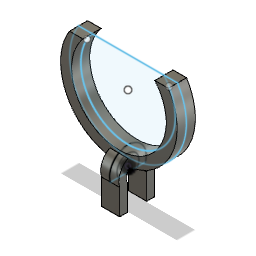
christmas-bell-door-clip-v6 (Autodesk Fusion 360 design; units mm, degrees)
Autodesk Fusion 360 part; units mm, degrees
sketch "Sketch1" plane through (0, 0, 0) normal (0, 0, 1) x (1, 0, 0)
  arc A0 (-11.2804, 24.5601) -> (11.2804, 24.5601) centre (0, 18.0985) ccw
  line L0 (13.5888, 26.545) -> (-13.5888, 26.545)
  arc A1 (-9.8821, 26.545) -> (9.8821, 26.545) centre (0, 18.0985) ccw
  arc A2 (-13.5888, 26.545) -> (13.5888, 26.545) centre (0, 18.0985) ccw
  dimension "d3" = 26
  dimension "d21" = 16
  constraint concentric A0 A1
  constraint horizontal L0
  constraint coincident L0 A1.end
  constraint coincident L0 A1.start
  measures "d3" diameter of A0
  measures "d21" radius of A2
extrude "Extrude1" add sketch "Sketch1" along normal mid plane 5 makes body 1
sketch "Sketch2" plane through (0, 0, 0) normal (1, 0, 0) x (0, 0, -1)
  line L0 (-4.783, -1.457) -> (4.783, -1.457)
  arc A0 (2.6224, -1.457) -> (-2.6224, -1.457) centre (0, 0) ccw
  arc A1 (4.783, -1.457) -> (-4.783, -1.457) centre (0, 0) ccw
  dimension "d9" = 3
  dimension "d10" = 5
  constraint horizontal L0
  constraint concentric A0 A1
  constraint coincident L0 A0.end
  constraint coincident L0 A0.start
  constraint coincident A0.centre A1.centre
  measures "d9" radius of A0
  measures "d10" radius of A1
extrude "Extrude2" add sketch "Sketch2" along normal mid plane 5 separate body contours L0 A0 A1 makes body 2
sketch "Sketch5" plane through (-2.5, 0, 0) normal (-1, 0, 0) x (0, 0, 1)
  line L0 (-4.783, -1.457) -> (-2.6224, -1.457)
  arc A0 (2.6224, -1.457) -> (-2.6224, -1.457) centre (0, 0) ccw
  line L1 (2.6224, -1.457) -> (4.783, -1.457)
  arc A1 (4.783, -1.457) -> (-4.783, -1.457) centre (0, 0) ccw
  line L2 (-2.506, 4.3267) -> (2.506, 4.3267)
  arc A2 (2.506, 4.3267) -> (-2.506, 4.3267) centre (0, 0) ccw
  constraint coincident A1 L2.start
  constraint coincident A1 L2.end
  constraint horizontal L2
extrude "Extrude3" cut sketch "Sketch5" against normal blind 5 contours A1 L2 A2 bodies 2
extrude "Extrude6" add 2 faces at (0.8333, -1.457, 3.3426) (-0.8333, -1.457, -3.3426) along direction (0, -1, 0) blind 7 on bodies 2 bodies 2
extrude "Extrude7" cut sketch "Sketch1" along normal mid plane 5 contours A0 L0 A1 bodies 1
extrude "Extrude9" cut sketch "Sketch2" along normal mid plane 20 contours L0 A0 bodies 1
